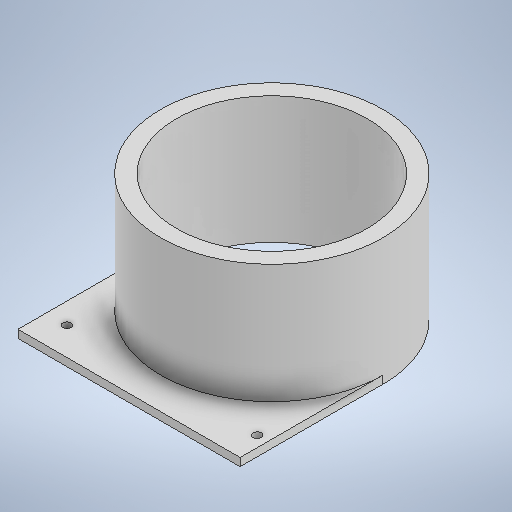
# Autodesk Inventor part: Battery_holder2
Saved by Autodesk Inventor 2025.3 (Build 293356000, 356)
## iProperties
Created: 2026-02-11
Part Number: Battery_holder2
Material: Generic
Document SubType Name: Modeling
Designer: m263126
Density: 1 g/cm^3
Appearance: Default
Author: m263126
Autodesk Inventor part; units mm, degrees
ref_plane "YZ Plane" through (0, 0, 0) normal (1, 0, 0) x (0, 1, 0)
ref_plane "XZ Plane" through (0, 0, 0) normal (0, 1, 0) x (-1, 0, 0)
ref_plane "XY Plane" through (0, 0, 0) normal (0, 0, 1) x (1, 0, 0)
sketch "Sketch1" plane through (0, 0, 0) normal (0, 1, 0) x (-1, 0, 0)
  circle A0 centre (0, 0) radius 38.1
  circle A1 centre (0, 0) radius 44.45
  dimension "d0" = 76.2
  dimension "d1" = 88.9
  constraints: 2 centre point, 2 coincident
  measures "d0" diameter of A0
  measures "d1" diameter of A1
sketch "Sketch2" plane through (0, 0, 0) normal (0, 1, 0) x (-1, 0, 0)
  circle A0 centre (0, 0) radius 44.45 projected
  line L0 (44.45, 0) -> (44.45, 57.15)
  line L1 (-44.45, 0) -> (-44.45, 57.15)
  line L2 (-44.45, 57.15) -> (44.45, 57.15)
  dimension "d8" = 57.15
  constraints: 6 end point, 2 point on circle, 2 vertical, 1 perpendicular, 1 tangent
  measures "d8" distance of L0.start L0.end
extrude "Extrusion1" add sketch "Sketch1" along normal blind 50.8
extrude "Extrusion2" add sketch "Sketch2" along normal blind 3.175
sketch "Sketch3" plane through (0, 3.175, 0) normal (0, 1, 0) x (1, 0, 0)
  circle A0 centre (0, 0) radius 38.1
  constraints: 1 centre point, 1 coincident
extrude "Extrusion3" cut sketch "Sketch3" against normal blind 3.175
sketch "Sketch4" plane through (0, 3.175, 0) normal (0, 1, 0) x (1, 0, 0)
  circle A0 centre (-36.068, -45.974) radius 1.6319
  line L0 (-44.45, 0) -> (-44.45, -57.15) projected
  line L1 (-44.45, -57.15) -> (44.45, -57.15) projected
  circle A1 centre (40.132, -45.974) radius 1.6319
  point P0 (0, 0)
  dimension "d11" = 3.2639
  dimension "d12" = 8.382
  dimension "d13" = 11.176
  dimension "d14" = 3.2639
  dimension "d15" = 76.2
  dimension "d16" = 0
  constraints: 2 centre point
  measures "d11" diameter of A0
  measures "d12" distance from line of L0 A0.centre
  measures "d13" distance from line of L1 A0.centre
  measures "d14" diameter of A1
  measures "d15" distance of A1.centre A0.centre
  measures "d16" vertical distance of A0.centre A1.centre
extrude "Extrusion4" cut sketch "Sketch4" against normal blind 3.175
body "Solid1"
